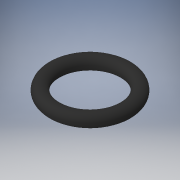
# Autodesk Inventor part: anel de borracha para m6
Saved by Autodesk Inventor 2019.4 (Build 234330000, 330)
## iProperties
Created: 2021-05-17
Part Number: anel de borracha para m6
Material: Borracha
Document SubType Name: Modeling
Designer: Lattes
Density: 0.93 g/cm^3
Appearance: Borracha - Preta
Author: Lattes
Autodesk Inventor part; units mm, degrees
ref_plane "YZ Plane" through (0, 0, 0) normal (1, 0, 0) x (0, 1, 0)
ref_plane "XZ Plane" through (0, 0, 0) normal (0, 1, 0) x (-1, 0, 0)
ref_plane "XY Plane" through (0, 0, 0) normal (0, 0, 1) x (1, 0, 0)
sketch "Esboço1" plane through (0, 0, 0) normal (0, 0, 1) x (1, 0, 0)
  line L0 (0, 0) -> (0, 13.919)
  line L1 (0, 0) -> (4, 0)
  line L2 (4, 0) -> (-4, 0)
  circle A0 centre (-4, 0) radius 0.75
  dimension "d0" = 4
  dimension "d1" = 8
  dimension "d2" = 1.5
  constraints: 6 end point, 2 horizontal, 1 centre point, 1 coincident, 1 vertical
  measures "d0" distance of L0.start L1.end
  measures "d1" distance of L1.end L2.end
  measures "d2" diameter of A0
revolve "Revolução1" add sketch "Esboço1" angle 360 about axis through (0, 0, 0) along (0, 1, 0)
